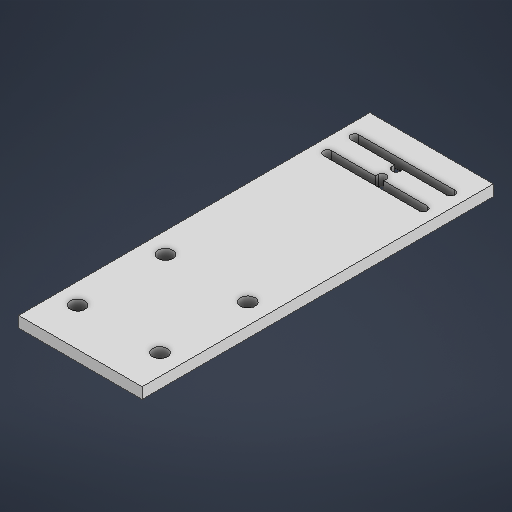
# Autodesk Inventor part: p2
Saved by Autodesk Inventor 2026 (Build 300175000, 175)
## iProperties
Created: 2025-04-19
Part Number: p2
Material: Generic
Document SubType Name: Modeling
Designer: jerem
Density: 1 g/cm^3
Appearance: Default
Author: jerem
## iProperties of the stored document p2_3DPrint.ipt
Created: 2025-04-19
Part Number: p2_3DPrint
Material: Generic
Document SubType Name: Modeling
Designer: jerem
Density: 1 g/cm^3
Appearance: Default
Author: jerem
Autodesk Inventor part; units mm, degrees
ref_plane "YZ Plane" through (0, 0, 0) normal (1, 0, 0) x (0, 1, 0)
ref_plane "XZ Plane" through (0, 0, 0) normal (0, 1, 0) x (-1, 0, 0)
ref_plane "XY Plane" through (0, 0, 0) normal (0, 0, 1) x (1, 0, 0)
sketch "Sketch1" plane through (0, 0, 0) normal (0, 1, 0) x (-1, 0, 0)
  line L0 (0, 0) -> (45, 0)
  line L1 (45, 0) -> (45, -128)
  line L2 (45, -128) -> (0, -128)
  line L3 (0, -128) -> (0, 0)
  line L4 (37.5, -14) -> (7.5, -14) construction
  line L5 (7.5, -14) -> (7.5, -46) construction
  line L6 (7.5, -46) -> (37.5, -46) construction
  line L7 (37.5, -46) -> (37.5, -14) construction
  circle A0 centre (37.5, -46) radius 2.7
  circle A1 centre (37.5, -14) radius 2.7
  circle A2 centre (7.5, -14) radius 2.7
  circle A3 centre (7.5, -46) radius 2.7
  line L8 (22.5, -14) -> (22.5, 0) construction
  circle A4 centre (5, -107.5) radius 1.5
  circle A5 centre (40, -107.5) radius 1.5
  line L9 (40, -109) -> (5, -109)
  line L10 (5, -106) -> (40, -106)
  line L11 (21, -109) -> (21, -116)
  line L12 (24, -116) -> (24, -109)
  line L13 (22.5, -116) -> (22.5, -109) construction
  circle A6 centre (40, -117.5) radius 1.5
  line L14 (5, -116) -> (40, -116)
  line L15 (40, -119) -> (5, -119)
  circle A7 centre (5, -117.5) radius 1.5
  line L16 (17.5, -109) -> (17.5, -116)
  line L17 (27.5, -116) -> (27.5, -109)
  line L18 (22.5, -116) -> (22.5, -128) construction
  line L19 (21, -111.5) -> (24, -111.5)
  line L20 (24, -113.5) -> (21, -113.5)
  point P0 (25, -109)
  point P1 (25, -116)
  point P2 (15, -116)
  point P3 (15, -109)
  point P4 (21.5, -116)
  point P5 (18.5, -116)
  point P6 (22.5, -112.5)
  point P7 (22.5, -111.5)
  dimension "d0" = 128
  dimension "d1" = 45
  dimension "d2" = 30
  dimension "d3" = 32
  dimension "d4" = 5.4
  dimension "d5" = 14
  dimension "d6" = 3
  dimension "d7" = 35
  dimension "d8" = 7
  dimension "d9" = 3
  dimension "d10" = 35
  dimension "d11" = 5
  dimension "d12" = 5
  dimension "d13" = 12
  dimension "d16" = 3
  dimension "d17" = 1.5
  dimension "d18" = 2
  dimension "d19" = 1
  constraints: 42 end point, 12 point on line, 8 centre point, 8 perpendicular, 8 point on circle, 8 tangent, 7 midpoint, 5 equal radius, 4 coincident, 4 horizontal, 4 parallel, 3 vertical
  measures "d0" distance of L0.end L1.end
  measures "d1" distance of L1.end L2.end
  measures "d2" distance of L6.end L5.end
  measures "d3" distance of L5.end L4.end
  measures "d4" diameter of A1
  measures "d5" distance between parallel lines of L0 L4
  measures "d6" diameter of A4
  measures "d7" distance of L10.start L10.end
  measures "d8" distance of L13.start L13.end
  measures "d9" diameter of A7
  measures "d10" distance of L14.start L14.end
  measures "d11" distance between parallel lines of L16 L13
  measures "d12" distance between parallel lines of L13 L17
  measures "d13" distance of L13.start L18.end
  measures "d16" distance between parallel lines of L12 L11
  measures "d17" distance between parallel lines of L13 L11
  measures "d18" distance between parallel lines of L20 L19
  measures "d19" distance of point (22.5, -112.5) point (22.5, -111.5)
extrude "Extrusion1" add sketch "Sketch1" along normal blind 4 contours L0 L1 L2 L3 | L9 L11 L14 L16 | L17 L14 L12 L9 | L19 L12 L20 L11
fillet "Fillet1" radius 1.5 4 edges at (-24, 2, -113.5) (-21, 2, -113.5) (-24, 2, -111.5) (-21, 2, -111.5)
equation "\"d12\" = d11"
equation "\"d17\" = 0.5 * d16"
equation "\"d19\" = 0.5 * d18"
body "Solid1"
